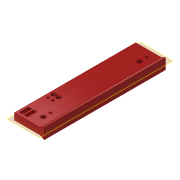
# Autodesk Inventor part: Front fixed bottom coupler
Saved by Autodesk Inventor 2020 (Build 240168000, 168)
## iProperties
Created: 2019-10-02
Part Number: Front fixed bottom coupler
Material: Generic
Document SubType Name: Modeling
Designer: ball
Density: 1 g/cm^3
Appearance: Default
Author: ball
Autodesk Inventor part; units mm, degrees
ref_plane "YZ Plane" through (0, 0, 0) normal (1, 0, 0) x (0, 1, 0)
ref_plane "XZ Plane" through (0, 0, 0) normal (0, 1, 0) x (-1, 0, 0)
ref_plane "XY Plane" through (0, 0, 0) normal (0, 0, 1) x (1, 0, 0)
sketch "Sketch1" plane through (0, 0, 0) normal (0, 1, 0) x (-1, 0, 0)
  line L0 (0, 0) -> (35.5, 0)
  line L1 (35.5, 0) -> (35.5, -170)
  line L2 (35.5, -170) -> (0, -170)
  line L3 (0, -170) -> (0, 0)
  dimension "d0" = 35.5
  dimension "d1" = 170
  constraints: 8 end point, 2 parallel, 1 horizontal, 1 perpendicular
  measures "d0" distance of L1.end L2.end
  measures "d1" distance of L0.end L1.end
extrude "Extrusion1" add sketch "Sketch1" along normal blind 9
sketch "Sketch2" plane through (0, 9, 0) normal (0, 1, 0) x (1, 0, 0)
  circle A0 centre (-10, 15) radius 3.25 construction
  line L0 (-35.5, 0) -> (0, 0) projected
  line L1 (0, 0) -> (0, 170) projected
  line L2 (-13.25, 15) -> (-11.625, 17.8146)
  line L3 (-11.625, 17.8146) -> (-8.375, 17.8146)
  line L4 (-8.375, 17.8146) -> (-6.75, 15)
  line L5 (-6.75, 15) -> (-8.375, 12.1854)
  line L6 (-8.375, 12.1854) -> (-11.625, 12.1854)
  line L7 (-11.625, 12.1854) -> (-13.25, 15)
  circle A1 centre (-10, 150) radius 3.25 construction
  line L8 (-13.25, 150) -> (-11.625, 152.8146)
  line L9 (-11.625, 152.8146) -> (-8.375, 152.8146)
  line L10 (-8.375, 152.8146) -> (-6.75, 150)
  line L11 (-6.75, 150) -> (-8.375, 147.1854)
  line L12 (-8.375, 147.1854) -> (-11.625, 147.1854)
  line L13 (-11.625, 147.1854) -> (-13.25, 150)
  line L14 (0, 170) -> (-35.5, 170) projected
  circle A2 centre (-10, 15) radius 1.7 construction
  circle A3 centre (-10, 150) radius 1.7 construction
  dimension "d7" = 6.5
  dimension "d10" = 6.5
  dimension "d23" = 135
  dimension "d24" = 15
  dimension "d25" = 10
  dimension "d28" = 3.4
  dimension "d29" = 3.4
  constraints: 24 end point, 4 coincident, 2 centre point, 2 horizontal alignment, 30 other
  measures "d23" distance of point (-10, 150) point (-10, 15)
  measures "d24" distance from line of L0 point (-10, 15)
  measures "d25" distance from line of L1 point (-10, 15)
  measures "d28" diameter of A2
  measures "d29" diameter of A3
extrude "Extrusion2" cut sketch "Sketch2" against normal blind 5
sketch "Sketch3" plane through (0, 0, 0) normal (0, -1, 0) x (1, 0, 0)
  circle A0 centre (-10, -25) radius 3.25 construction
  line L0 (0, 0) -> (-35.5, 0) projected
  line L1 (-35.5, 0) -> (-35.5, -170) projected
  line L2 (-11.6286, -27.8125) -> (-13.25, -24.9958)
  line L3 (-13.25, -24.9958) -> (-11.6214, -22.1833)
  line L4 (-11.6214, -22.1833) -> (-8.3714, -22.1875)
  line L5 (-8.3714, -22.1875) -> (-6.75, -25.0042)
  line L6 (-6.75, -25.0042) -> (-8.3786, -27.8167)
  line L7 (-8.3786, -27.8167) -> (-11.6286, -27.8125)
  circle A1 centre (-10, -160) radius 3.25 construction
  line L8 (-6.75, -160) -> (-8.375, -162.8146)
  line L9 (-8.375, -162.8146) -> (-11.625, -162.8146)
  line L10 (-11.625, -162.8146) -> (-13.25, -160)
  line L11 (-13.25, -160) -> (-11.625, -157.1854)
  line L12 (-11.625, -157.1854) -> (-8.375, -157.1854)
  line L13 (-8.375, -157.1854) -> (-6.75, -160)
  line L14 (0, -170) -> (0, 0) projected
  dimension "d15" = 6.5
  dimension "d18" = 6.5
  dimension "d16" = 25
  dimension "d19" = 135
  dimension "d26" = 10
  dimension "d27" = 10
  constraints: 24 end point, 2 coincident, 1 horizontal alignment, 31 other
  measures "d16" distance from line of L0 point (-10, -25)
  measures "d19" distance of point (-10, -160) point (-10, -25)
  measures "d26" distance from line of L14 point (-10, -25)
  measures "d27" distance from line of L14 point (-10, -160)
extrude "Extrusion3" cut sketch "Sketch3" against normal blind 5
sketch "Sketch5" plane through (0, 9, 0) normal (0, 1, 0) x (1, 0, 0)
  circle A0 centre (-10, 15) radius 1.7
  line L0 (0, 0) -> (0, 170) projected
  line L1 (-35.5, 0) -> (0, 0) projected
  circle A1 centre (-10, 150) radius 1.7
  circle A2 centre (-10, 25) radius 1.7
  circle A3 centre (-10, 160) radius 1.7
  dimension "d30" = 3.4
  dimension "d31" = 10
  dimension "d32" = 15
  dimension "d33" = 3.4
  dimension "d34" = 10
  dimension "d35" = 135
  dimension "d36" = 3.4
  dimension "d37" = 25
  dimension "d38" = 3.4
  dimension "d39" = 10
  dimension "d40" = 135
  constraints: 4 centre point
  measures "d30" diameter of A0
  measures "d31" distance from line of L0 A0.centre
  measures "d32" distance from line of L1 A0.centre
  measures "d33" diameter of A1
  measures "d34" distance from line of L0 A1.centre
  measures "d35" distance of A1.centre A0.centre
  measures "d36" diameter of A2
  measures "d37" distance from line of L1 A2.centre
  measures "d38" diameter of A3
  measures "d39" distance from line of L0 A3.centre
  measures "d40" distance of A2.centre A3.centre
extrude "Extrusion4" cut sketch "Sketch5" against normal through all
sketch "Sketch6" plane through (0, 9, 0) normal (0, 1, 0) x (1, 0, 0)
  line L0 (-32.5, 4) -> (-27.7502, 4)
  line L1 (-27.7502, 4) -> (-27.7502, 16.7)
  line L2 (-27.7502, 16.7) -> (-32.5, 16.7)
  line L3 (-32.5, 16.7) -> (-32.5, 4)
  line L4 (-35.5, 0) -> (0, 0) projected
  line L5 (-35.5, 170) -> (-35.5, 0) projected
  line L6 (-25.7502, 4) -> (-21.0002, 4)
  line L7 (-21.0002, 4) -> (-21.0002, 16.7)
  line L8 (-21.0002, 16.7) -> (-25.7502, 16.7)
  line L9 (-25.7502, 16.7) -> (-25.7502, 4)
  line L10 (0, 0) -> (0, 170) construction
  line L11 (-35.5, 170) -> (0, 170) projected
  line L12 (0, 0) -> (-20, 0) construction
  line L13 (-20, 0) -> (-20, 170) construction
  line L14 (-20, 170) -> (0, 170) construction
  line L15 (0, 170) -> (0, 0)
  circle A0 centre (-23.3752, 41.7) radius 1.7
  circle A1 centre (-30.125, 41.7) radius 1.7
  circle A2 centre (-30.125, 49.7) radius 1.7
  circle A3 centre (-23.3752, 49.7) radius 1.7
  dimension "d43" = 4.7498
  dimension "d44" = 12.7
  dimension "d45" = 4
  dimension "d46" = 3
  dimension "d47" = 4.75
  dimension "d48" = 2
  dimension "d49" = 20
  dimension "d50" = 3.4
  dimension "d51" = 25
  dimension "d87" = 3.4
  dimension "d88" = 5.375
  dimension "d90" = 3.4
  dimension "d91" = 8
  dimension "d92" = 3.4
  constraints: 24 end point, 6 parallel, 4 centre point, 3 horizontal, 3 perpendicular, 1 point on line
  measures "d43" distance of L2.end L1.end
  measures "d44" distance of L1.end L0.end
  measures "d45" distance between parallel lines of L4 L0
  measures "d46" distance between parallel lines of L5 L3
  measures "d47" distance of L8.end L7.end
  measures "d48" distance between parallel lines of L9 L1
  measures "d49" distance of L13.end L14.end
  measures "d50" diameter of A0
  measures "d51" distance from line of A0.centre L8
  measures "d87" diameter of A1
  measures "d88" distance from line of L5 A1.centre
  measures "d90" diameter of A2
  measures "d91" distance of A2.centre A1.centre
  measures "d92" diameter of A3
extrude "Extrusion5" cut sketch "Sketch6" against normal through all contours L3 L2 L1 L0 | L9 L8 L7 L6 | A0 | A1 | A2 | A3
sketch "Sketch7" plane through (0, 0, 0) normal (0, -1, 0) x (1, 0, 0)
  circle A0 centre (-23.3752, -41.7) radius 1.7 projected
  circle A1 centre (-23.3752, -41.7) radius 3.25 construction
  line L0 (-23.3752, -38.45) -> (-20.5606, -40.075)
  line L1 (-20.5606, -40.075) -> (-20.5606, -43.325)
  line L2 (-20.5606, -43.325) -> (-23.3752, -44.95)
  line L3 (-23.3752, -44.95) -> (-26.1898, -43.325)
  line L4 (-26.1898, -43.325) -> (-26.1898, -40.075)
  line L5 (-26.1898, -40.075) -> (-23.3752, -38.45)
  circle A2 centre (-30.1625, -41.7) radius 3.25 construction
  line L6 (-30.125, -38.4502) -> (-27.3294, -40.1076)
  line L7 (-27.3294, -40.1076) -> (-27.3669, -43.3574)
  line L8 (-27.3669, -43.3574) -> (-30.2, -44.9498)
  line L9 (-30.2, -44.9498) -> (-32.9956, -43.2924)
  line L10 (-32.9956, -43.2924) -> (-32.9581, -40.0426)
  line L11 (-32.9581, -40.0426) -> (-30.125, -38.4502)
  point P0 (0, 0)
  dimension "d89" = 6.5
  dimension "d54" = 6.5
  constraints: 24 end point, 3 coincident, 1 centre point, 17 other
  measures "d54" diameter of A1
extrude "Extrusion6" cut sketch "Sketch7" against normal blind 5
sketch "Sketch8" plane through (-35.5, 0, -170) normal (-1, 0, 0) x (0, 0, 1)
  circle A0 centre (159.65, 4.5) radius 1.4605
  line L0 (0, 9) -> (170, 9) projected
  line L1 (170, 0) -> (170, 9) projected
  dimension "d57" = 2.921
  dimension "d58" = 4.5
  dimension "d59" = 10.35
  constraints: 1 centre point
  measures "d57" diameter of A0
  measures "d58" distance from line of L0 A0.centre
  measures "d59" distance from line of L1 A0.centre
hole "Hole1" at (-35.5, 4.5, -10.35) direction (1, 0, 0) diameter 2.921 depth 21 counterbore diameter 3.4 counterbore depth 1.5
sketch "Sketch9" plane through (-21.0002, 9, -16.7) normal (-1, 0, 0) x (0, 0, 1)
  circle A0 centre (6.35, -4.5) radius 1.4605 projected
  circle A1 centre (6.35, -4.5) radius 2.54
  point P0 (16.7, -9)
  dimension "d67" = 5.08
  constraints: 1 centre point, 1 coincident
  measures "d67" diameter of A1
extrude "Extrusion7" add sketch "Sketch9" along normal blind 0.2032
sketch "Sketch10" plane through (-27.7502, 9, -16.7) normal (-1, 0, 0) x (0, 0, 1)
  circle A0 centre (6.35, -4.5) radius 1.7 projected
  circle A1 centre (6.35, -4.5) radius 2.54
  point P0 (16.7, -9)
  dimension "d70" = 5.08
  constraints: 1 centre point, 1 coincident
  measures "d70" diameter of A1
extrude "Extrusion8" add sketch "Sketch10" along normal blind 0.2032
sketch "Sketch11" plane through (-25.7502, 9, -4) normal (1, 0, 0) x (0, 0, -1)
  circle A0 centre (6.35, -4.5) radius 1.7 projected
  circle A1 centre (6.35, -4.5) radius 2.54
  point P0 (-4, -9)
  dimension "d73" = 5.08
  constraints: 1 centre point, 1 coincident
  measures "d73" diameter of A1
extrude "Extrusion9" add sketch "Sketch11" along normal blind 0.2032
sketch "Sketch12" plane through (-32.5, 9, -4) normal (1, 0, 0) x (0, 0, -1)
  circle A0 centre (6.35, -4.5) radius 1.7 projected
  circle A1 centre (6.35, -4.5) radius 2.54
  point P0 (-4, -9)
  dimension "d76" = 5.08
  constraints: 1 centre point, 1 coincident
  measures "d76" diameter of A1
extrude "Extrusion10" add sketch "Sketch12" along normal blind 0.2032
sketch "Sketch14" plane through (0, 0, -170) normal (0, 0, -1) x (-1, 0, 0)
  circle A0 centre (18, 4.5) radius 2.25
  line L0 (35.5, 0) -> (0, 0) projected
  line L1 (0, 0) -> (0, 9) projected
  dimension "d82" = 4.5
  dimension "d83" = 4.5
  dimension "d84" = 18
  constraints: 1 centre point
  measures "d82" diameter of A0
  measures "d83" distance from line of L0 A0.centre
  measures "d84" distance from line of L1 A0.centre
extrude "Extrusion11" cut sketch "Sketch14" against normal blind 71
sketch "Sketch15" plane through (0, 9, 0) normal (0, 1, 0) x (1, 0, 0)
  circle A0 centre (-30.125, 49.7) radius 1.7 projected
  circle A1 centre (-30.125, 49.7) radius 3.25 construction
  circle A2 centre (-23.3752, 49.7) radius 1.7 projected
  circle A3 centre (-23.3752, 49.7) radius 3.25 construction
  line L0 (-30.125, 46.45) -> (-32.9396, 48.075)
  line L1 (-32.9396, 48.075) -> (-32.9396, 51.325)
  line L2 (-32.9396, 51.325) -> (-30.125, 52.95)
  line L3 (-30.125, 52.95) -> (-27.3104, 51.325)
  line L4 (-27.3104, 51.325) -> (-27.3104, 48.075)
  line L5 (-27.3104, 48.075) -> (-30.125, 46.45)
  line L6 (-23.3752, 46.45) -> (-26.1898, 48.075)
  line L7 (-26.1898, 48.075) -> (-26.1898, 51.325)
  line L8 (-26.1898, 51.325) -> (-23.3752, 52.95)
  line L9 (-23.3752, 52.95) -> (-20.5606, 51.325)
  line L10 (-20.5606, 51.325) -> (-20.5606, 48.075)
  line L11 (-20.5606, 48.075) -> (-23.3752, 46.45)
  point P0 (0, 0)
  dimension "d93" = 6.5
  dimension "d94" = 6.5
  constraints: 24 end point, 4 coincident, 2 vertical alignment, 30 other
extrude "Extrusion12" cut sketch "Sketch15" against normal blind 5
sketch "Sketch17" plane through (-35.5, 0, 0) normal (0, 0, 1) x (1, 0, 0)
  line L0 (0, 9) -> (35.5, 9) projected
  line L1 (35.5, 0) -> (35.5, 9) projected
  line L2 (35.5, 9) -> (35.754, 9)
  line L3 (35.754, 0) -> (35.5, 0)
  line L4 (35.5, 0) -> (35.5, 9)
  line L5 (41.85, 12.048) -> (41.85, -3.048)
  line L6 (35.754, 9) -> (41.85, 12.048)
  line L7 (35.754, 0) -> (41.85, -3.048)
  dimension "d100" = 0.254
  dimension "d107" = 3.048
  dimension "d109" = 3.048
  dimension "d110" = 15.096
  dimension "d111" = 0.254
  constraints: 12 end point, 1 horizontal, 1 parallel
  measures "d100" distance of L3.start L3.end
  measures "d107" vertical distance of L5.start L2.end
  measures "d109" vertical distance of L3.start L5.end
  measures "d110" distance of L5.start L5.end
  measures "d111" distance of L0.end L2.end
extrude "SLiding Insert" add sketch "Sketch17" against normal up to surface (170 mm away)
sketch "Sketch18" plane through (-32.5, 9, -4) normal (1, 0, 0) x (0, 0, -1)
  line L0 (12.7, -9) -> (0, -9) construction
  line L1 (0, 0) -> (0, -9) construction
  line L2 (12.7, -9) -> (0, -9) construction
  line L3 (0, -9) -> (0, 0) construction
  line L4 (0, 0) -> (12.7, 0) construction
  line L5 (12.7, 0) -> (12.7, -9) construction
  line L6 (166, 0) -> (-4, 0) projected
  line L7 (-4, -9) -> (166, -9) projected
  line L8 (3.175, 0) -> (3.556, 0)
  line L9 (3.556, 0) -> (3.556, -9)
  line L10 (3.556, -9) -> (3.175, -9)
  line L11 (3.175, -9) -> (3.175, 0)
  line L12 (9.525, 0) -> (9.144, 0)
  line L13 (9.144, 0) -> (9.144, -9)
  line L14 (9.144, -9) -> (9.525, -9)
  line L15 (9.525, -9) -> (9.525, 0)
  line L16 (6.35, 0) -> (6.731, 0)
  line L17 (6.731, 0) -> (6.731, -9)
  line L18 (6.731, -9) -> (6.35, -9)
  line L19 (6.35, -9) -> (6.35, 0)
  point P0 (9.144, 0)
  point P1 (9.144, -9)
  point P2 (6.35, 0)
  point P3 (6.731, 0)
  dimension "d114" = 0.381
  dimension "d115" = 0.381
  dimension "d116" = 0.381
  dimension "d117" = 3.175
  dimension "d118" = 3.175
  dimension "d120" = 6.35
  constraints: 32 end point, 8 parallel, 5 point on line, 4 horizontal, 4 perpendicular
  measures "d114" distance of L9.end L10.end
  measures "d115" distance of L14.end L13.end
  measures "d116" distance of L17.end L18.end
  measures "d117" distance of L10.end L0.end
  measures "d118" distance of L0.start L14.end
  measures "d120" distance of L18.end L0.end
extrude "Supports 1" add sketch "Sketch18" along normal up to surface (4.7498 mm away) contours L15 L7 L13 L6 | L17 L7 L19 L6 | L9 L7 L11 L6
sketch "Sketch19" plane through (-25.7502, 9, -4) normal (1, 0, 0) x (0, 0, -1)
  line L0 (12.7, 0) -> (0, 0) construction
  line L1 (0, 0) -> (0, -9) construction
  line L2 (0, -9) -> (12.7, -9) construction
  line L3 (12.7, -9) -> (12.7, 0) construction
  line L4 (6.731, 0) -> (6.731, -1.9887) projected
  line L5 (6.731, 0) -> (6.35, 0)
  line L6 (6.35, 0) -> (6.35, -9)
  line L7 (6.35, -9) -> (6.731, -9)
  line L8 (6.731, -9) -> (6.731, 0)
  line L9 (9.525, 0) -> (9.525, -9) projected
  line L10 (6.731, -9) -> (9.144, -9) projected
  line L11 (9.525, 0) -> (9.144, 0)
  line L12 (9.144, 0) -> (9.144, -9)
  line L13 (9.144, -9) -> (9.525, -9)
  line L14 (9.525, -9) -> (9.525, 0)
  line L15 (3.175, 0) -> (0, 0) projected
  line L16 (3.556, 0) -> (3.556, -9) projected
  line L17 (3.175, 0) -> (3.556, 0)
  line L18 (3.556, 0) -> (3.556, -9)
  line L19 (3.556, -9) -> (3.175, -9)
  line L20 (3.175, -9) -> (3.175, 0)
  point P0 (-4, -9)
  constraints: 32 end point, 8 parallel, 4 horizontal, 4 perpendicular, 1 midpoint
extrude "Supports 2" add sketch "Sketch19" along normal up to surface (4.75 mm away)
ref_plane "Work Plane1" through (-30.1251, 9, -7.556) normal (1, 0, 0) x (0, 0, -1)
ref_plane "Work Plane2" through (-23.3752, 0, -4) normal (1, 0, 0) x (0, 0, -1)
ref_plane "Work Plane3" through (0, 4.5, 0) normal (0, 1, 0) x (1, 0, 0)
equation "\"d109\" = d107"
equation "\"d111\" = d100"
equation "\"d118\" = d117"
body "Solid1"
